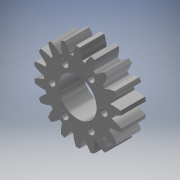
# Autodesk Inventor part: Цилиндрическое зубчатое зацепление2
Saved by Autodesk Inventor 2019 (Build 230136000, 136)
## iProperties
Created: 2020-03-13
Part Number: Цилиндрическое зубчатое зацепление2
Material: Steel
Document SubType Name: Modeling
Designer: Петров Иван
Categories: <?xml version="1.0" encoding="UTF-16"?> <MemberInstance><Categories><FamilyTemplate><FamilyTemplateParameter ValueType="xs:double" Id="1" ObjectReferenceKey="da_z" ObjectType="kUserParameterObject"/><FamilyTemplateParameter ValueType="xs:double" Id="2" ObjectReferenceKey="da_b" ObjectType="kUserParameterObject"/><FamilyTemplateParameter ValueType="xs:double" Id="3" ObjectReferenceKey="da_beta" ObjectType="kUserParameterObject"/><FamilyTemplateParameter ValueType="xs:double" Id="4" ObjectReferenceKey="da_da" ObjectType="kUserParameterObject"/><FamilyTemplateParameter ValueType="xs:double" Id="5" ObjectReferenceKey="da_aw" ObjectType="kUserParameterObject"/><FamilyTemplateParameter ValueType="xs:string" Id="6" ObjectReferenceKey="EAIAABAAAACIAQAAAAAAAIAAAAAAAAAA" ObjectType="83910656" SubObjectId="SurfaceGeometry"/></FamilyTemplate><ParamToTemplateMap><ParamToTemplate CategoryParameter="//CategoryParameter[@InternalName='046C89C9-8512-4d59-83FE-43B91F4F132A']" TemplateParameter="1"/><ParamToTemplate CategoryParameter="//CategoryParameter[@InternalName='2552DF32-E462-4b46-AEBF-C6C7768E72AC']" TemplateParameter="2"/><ParamToTemplate CategoryParameter="//CategoryParameter[@InternalName='C9EE641D-15FC-4fae-A226-E94C4372FDD7']" TemplateParameter="3"/><ParamToTemplate><ParamToTemplate CategoryParameter="//CategoryParameter[@InternalName='00B6519A-459B-49c7-AD84-2E56D39A5744']" ConstantValue="-0.108464"/></ParamToTemplate><ParamToTemplate><ParamToTemplate CategoryParameter="//CategoryParameter[@InternalName='04B31F0E-C7A6-4894-AA32-9629BEFACF47']" ConstantValue="1.000000"/></ParamToTemplate><ParamToTemplate><ParamToTemplate CategoryParameter="//CategoryParameter[@InternalName='43CBEC2E-7847-49e7-A936-2F7889FCB2D9']" ConstantValue="0.250000"/></ParamToTemplate><ParamToTemplate><ParamToTemplate CategoryParameter="//CategoryParameter[@InternalName='B1EFC894-105D-4ebd-86BF-FA20ED196853']" ConstantValue="0.350000"/></ParamToTemplate><ParamToTemplate><ParamToTemplate CategoryParameter="//CategoryParameter[@InternalName='51175063-3D10-4879-93E8-6246FE8B403D']" ConstantValue="2060000000.000000"/></ParamToTemplate><ParamToTemplate><ParamToTemplate CategoryParameter="//CategoryParameter[@InternalName='A3A52E27-4454-46a9-B0BD-C932399B70AF']" ConstantValue="0.300000"/></ParamToTemplate><ParamToTemplate><ParamToTemplate CategoryParameter="//CategoryParameter[@InternalName='91B76062-C214-41d9-B1B9-14D2AB99603D']" ConstantValue="0.090000"/></ParamToTemplate><ParamToTemplate><ParamToTemplate CategoryParameter="//CategoryParameter[@InternalName='374E806E-8B8A-4dda-A9AA-1039D6500AD2']" ConstantValue="11.111111"/></ParamToTemplate><ParamToTemplate><ParamToTemplate CategoryParameter="//CategoryParameter[@InternalName='2D373A89-B862-43d6-8D0B-0CBF12AB9F6C']" ConstantValue="0.349066"/></ParamToTemplate><ParamToTemplate CategoryParameter="//CategoryParameter[@InternalName='37777632-D6A2-4fac-9D53-DB8ACD95C989']" TemplateParameter="4"/><ParamToTemplate CategoryParameter="//CategoryParameter[@InternalName='FD1017F1-B727-4f7e-9707-0F86F1FF9423']" TemplateParameter="5"/><ParamToTemplate><ParamToTemplate CategoryParameter="//CategoryParameter[@InternalName='9E1B4470-B2D3-4ff1-B813-535BB4CDF51A']" ConstantValue="3520000.000000"/></ParamToTemplate><ParamToTemplate><ParamToTemplate CategoryParameter="//CategoryParameter[@InternalName='F8452263-BFF6-458c-9FB1-07C4B99E95CD']" ConstantValue="11400000.000000"/></ParamToTemplate><ParamToTemplate><ParamToTemplate CategoryParameter="//CategoryParameter[@InternalName='3E3BB259-FD49-497f-8171-6EBC954A3479']" ConstantValue="2.000000"/></ParamToTemplate><ParamToTemplate CategoryParameter="//CategoryParameter[@InternalName='27C3BAF2-7550-4e4b-AE2C-0DB134B7D9B7']" TemplateParameter="6"/></ParamToTemplateMap><Category DisplayName="Gear" InternalName="DC85795E-93AB-48d5-8EEE-5A27447B64BD" Mnemonic="Gear"><CategoryParameter DisplayName="z" InternalName="046C89C9-8512-4d59-83FE-43B91F4F132A" Mnemonic="z"/><CategoryParameter DisplayName="b" InternalName="2552DF32-E462-4b46-AEBF-C6C7768E72AC" Mnemonic="b"/><CategoryParameter DisplayName="||b|" InternalName="C9EE641D-15FC-4fae-A226-E94C4372FDD7" Mnemonic="beta"/><CategoryParameter DisplayName="x" InternalName="00B6519A-459B-49c7-AD84-2E56D39A5744" Mnemonic="x"/><CategoryParameter DisplayName="a*" InternalName="04B31F0E-C7A6-4894-AA32-9629BEFACF47" Mnemonic="a"/><CategoryParameter DisplayName="c*" InternalName="43CBEC2E-7847-49e7-A936-2F7889FCB2D9" Mnemonic="c"/><CategoryParameter DisplayName="r|.f|*" InternalName="B1EFC894-105D-4ebd-86BF-FA20ED196853" Mnemonic="rf"/><CategoryParameter DisplayName="E" InternalName="51175063-3D10-4879-93E8-6246FE8B403D" Mnemonic="E"/><CategoryParameter DisplayName="||m|" InternalName="A3A52E27-4454-46a9-B0BD-C932399B70AF" Mnemonic="mi"/><Category DisplayName="SpurGear" InternalName="26C5A22E-A91E-4dfd-A3B3-23CCAFAE1764" Mnemonic="SpurGear"><CategoryParameter DisplayName="m" InternalName="91B76062-C214-41d9-B1B9-14D2AB99603D" Mnemonic="m"/><CategoryParameter DisplayName="P" InternalName="374E806E-8B8A-4dda-A9AA-1039D6500AD2" Mnemonic="PP"/><CategoryParameter DisplayName="||a|" InternalName="2D373A89-B862-43d6-8D0B-0CBF12AB9F6C" Mnemonic="alpha"/><CategoryParameter DisplayName="d|.a|" InternalName="37777632-D6A2-4fac-9D53-DB8ACD95C989" Mnemonic="da"/><CategoryParameter DisplayName="a|.w|" InternalName="FD1017F1-B727-4f7e-9707-0F86F1FF9423" Mnemonic="aw"/><CategoryParameter DisplayName="||s||.Flim|" InternalName="9E1B4470-B2D3-4ff1-B813-535BB4CDF51A" Mnemonic="sFlim"/><CategoryParameter DisplayName="||s||.Hlim|" InternalName="F8452263-BFF6-458c-9FB1-07C4B99E95CD" Mnemonic="sHlim"/><CategoryParameter DisplayName="тип" InternalName="3E3BB259-FD49-497f-8171-6EBC954A3479" Mnemonic="type"/><CategoryParameter DisplayName="PitchDiameter" InternalName="27C3BAF2-7550-4e4b-AE2C-0DB134B7D9B7" Mnemonic="IDS_PITCHDIAM"/></Category></Category></Categories></MemberInstance>
Density: 1 g/cm^3
Appearance: Steel
CustomPartVersion: 1
Author: Петров Иван
Autodesk Inventor part; units mm, degrees
ref_plane "YZ Plane" through (0, 0, 0) normal (1, 0, 0) x (0, 1, 0)
ref_plane "XZ Plane" through (0, 0, 0) normal (0, 1, 0) x (-1, 0, 0)
ref_plane "XY Plane" through (0, 0, 0) normal (0, 0, 1) x (1, 0, 0)
sketch "Sketch1" plane through (0, 0, 0) normal (0, 0, 1) x (1, 0, 0)
  circle A0 centre (0, 0) radius 8.9
  dimension "d0" = 17.8
  constraints: 1 centre point
  measures "d0" diameter of A0
extrude "Extrusion1" add sketch "Sketch1" along normal blind 5
ref_plane "Work Plane2" through (0, 0, 2.5) normal (0, 0, 1) x (1, 0, 0)
sketch "Sketch2" plane through (0, 0, 0) normal (0, 0, -1) x (-1, 0, 0)
  circle A0 centre (0, 0) radius 8.9 projected
  circle A1 centre (0, 0) radius 8.05
  dimension "d3" = 16.1
  constraints: 1 centre point, 1 coincident
  measures "d3" diameter of A1
surface extrude "Средний диаметр" sketch "Sketch2" against normal through all shown no curves A1
ref_plane "Work Plane8" through (0, 0, 0) normal (0.9848078, 0.1736482, 0) x (0, 0, 1)
ref_plane "Work Plane9" through (0, 0, 0) normal (1, 0, 0) x (0, 1, 0)
spur gear teeth "Цилиндрическое зубчатое зацепление" teeth 18 pitch diameter 16.2 tip diameter 17.8 root diameter 13.7548 face width 5 start plane through (0, 0, 0) normal (0, 0, -1) x (-1, 0, 0)
sketch "Эскиз3" plane through (0, 0, 5) normal (0, 0, 1) x (1, 0, 0)
  circle A0 centre (0, 0) radius 3.85
  dimension "d49" = 7.7
  constraints: 1 centre point, 1 coincident
  measures "d49" diameter of A0
extrude "Выдавливание2" cut sketch "Эскиз3" against normal blind 12
sketch "Эскиз4" plane through (0, 0, 5) normal (0, 0, 1) x (1, 0, 0)
  line L0 (0, 0) -> (-5.3, 0)
  circle A0 centre (-5.3, 0) radius 0.75
  dimension "d52" = 5.3
  dimension "d53" = 1.5
  constraints: 2 end point, 1 centre point, 1 coincident, 1 horizontal
  measures "d52" distance of L0.start L0.end
  measures "d53" diameter of A0
extrude "Выдавливание3" cut sketch "Эскиз4" against normal blind 33.25
pattern_circular "Круговой массив1" count 6 over 360 about axis through (0, 0, 5) along (0, 0, -1) of "Выдавливание3"
sketch "Эскиз5" plane through (0, 0, 5) normal (0, 0, 1) x (1, 0, 0)
  circle A0 centre (-2.65, -4.5899) radius 0.75 projected
  circle A1 centre (2.65, -4.5899) radius 0.75 projected
  circle A2 centre (5.3, 0) radius 0.75 projected
  circle A3 centre (2.65, 4.5899) radius 0.75 projected
  circle A4 centre (-2.65, 4.5899) radius 0.75 projected
  circle A5 centre (-5.3, 0) radius 0.75 projected
  circle A6 centre (0, 0) radius 3.85 projected
  arc A7 (-3.4059, 8.2225) -> (-3.1756, 6.1003) centre (3.6513, 7.9146) ccw projected
  arc A8 (-3.1756, 6.1003) -> (-3.6952, 5.8003) centre (0, 0) ccw projected
  arc A9 (-3.6952, 5.8003) -> (-5.418, 7.0608) centre (-8.6799, 0.7952) ccw projected
  arc A10 (-5.418, 7.0608) -> (-6.0128, 6.5618) centre (0, 0) ccw projected
  arc A11 (-6.0128, 6.5618) -> (-5.0705, 4.6463) centre (0.7241, 8.6861) ccw projected
  arc A12 (-5.0705, 4.6463) -> (-5.4562, 4.1867) centre (0, 0) ccw projected
  arc A13 (-5.4562, 4.1867) -> (-7.5062, 4.782) centre (-8.4284, -2.2214) ccw projected
  arc A14 (-7.5062, 4.782) -> (-7.8944, 4.1096) centre (0, 0) ccw projected
  arc A15 (-7.8944, 4.1096) -> (-6.3539, 2.6319) centre (-2.2904, 8.4099) ccw projected
  arc A16 (-6.3539, 2.6319) -> (-6.5591, 2.0681) centre (0, 0) ccw projected
  arc A17 (-6.5591, 2.0681) -> (-8.689, 1.9263) centre (-7.1604, -4.9702) ccw projected
  arc A18 (-8.689, 1.9263) -> (-8.8239, 1.1617) centre (0, 0) ccw projected
  arc A19 (-8.8239, 1.1617) -> (-6.8708, 0.3) centre (-5.0286, 7.1194) ccw projected
  arc A20 (-6.8708, 0.3) -> (-6.8708, -0.3) centre (0, 0) ccw projected
  arc A21 (-6.8708, -0.3) -> (-8.8239, -1.1617) centre (-5.0286, -7.1194) ccw projected
  arc A22 (-8.8239, -1.1617) -> (-8.689, -1.9263) centre (0, 0) ccw projected
  arc A23 (-8.689, -1.9263) -> (-6.5591, -2.0681) centre (-7.1604, 4.9702) ccw projected
  arc A24 (-6.5591, -2.0681) -> (-6.3539, -2.6319) centre (0, 0) ccw projected
  arc A25 (-6.3539, -2.6319) -> (-7.8944, -4.1096) centre (-2.2904, -8.4099) ccw projected
  arc A26 (-7.8944, -4.1096) -> (-7.5062, -4.782) centre (0, 0) ccw projected
  arc A27 (-7.5062, -4.782) -> (-5.4562, -4.1867) centre (-8.4284, 2.2214) ccw projected
  arc A28 (-5.4562, -4.1867) -> (-5.0705, -4.6463) centre (0, 0) ccw projected
  arc A29 (-5.0705, -4.6463) -> (-6.0128, -6.5618) centre (0.7241, -8.6861) ccw projected
  arc A30 (-6.0128, -6.5618) -> (-5.418, -7.0608) centre (0, 0) ccw projected
  arc A31 (-5.418, -7.0608) -> (-3.6952, -5.8003) centre (-8.6799, -0.7952) ccw projected
  arc A32 (-3.6952, -5.8003) -> (-3.1756, -6.1003) centre (0, 0) ccw projected
  arc A33 (-3.1756, -6.1003) -> (-3.4059, -8.2225) centre (3.6513, -7.9146) ccw projected
  arc A34 (-3.4059, -8.2225) -> (-2.6763, -8.4881) centre (0, 0) ccw projected
  arc A35 (-2.6763, -8.4881) -> (-1.4885, -6.7144) centre (-7.8845, -3.716) ccw projected
  arc A36 (-1.4885, -6.7144) -> (-0.8977, -6.8185) centre (0, 0) ccw projected
  arc A37 (-0.8977, -6.8185) -> (-0.3882, -8.8915) centre (6.138, -6.1885) ccw projected
  arc A38 (-0.3882, -8.8915) -> (0.3882, -8.8915) centre (0, 0) ccw projected
  arc A39 (0.3882, -8.8915) -> (0.8977, -6.8185) centre (-6.138, -6.1885) ccw projected
  arc A40 (0.8977, -6.8185) -> (1.4885, -6.7144) centre (0, 0) ccw projected
  arc A41 (1.4885, -6.7144) -> (2.6763, -8.4881) centre (7.8845, -3.716) ccw projected
  arc A42 (2.6763, -8.4881) -> (3.4059, -8.2225) centre (0, 0) ccw projected
  arc A43 (3.4059, -8.2225) -> (3.1756, -6.1003) centre (-3.6513, -7.9146) ccw projected
  arc A44 (3.1756, -6.1003) -> (3.6952, -5.8003) centre (0, 0) ccw projected
  arc A45 (3.6952, -5.8003) -> (5.418, -7.0608) centre (8.6799, -0.7952) ccw projected
  arc A46 (5.418, -7.0608) -> (6.0128, -6.5618) centre (0, 0) ccw projected
  arc A47 (6.0128, -6.5618) -> (5.0705, -4.6463) centre (-0.7241, -8.6861) ccw projected
  arc A48 (5.0705, -4.6463) -> (5.4562, -4.1867) centre (0, 0) ccw projected
  arc A49 (5.4562, -4.1867) -> (7.5062, -4.782) centre (8.4284, 2.2214) ccw projected
  arc A50 (7.5062, -4.782) -> (7.8944, -4.1096) centre (0, 0) ccw projected
  arc A51 (7.8944, -4.1096) -> (6.3539, -2.6319) centre (2.2904, -8.4099) ccw projected
  arc A52 (6.3539, -2.6319) -> (6.5591, -2.0681) centre (0, 0) ccw projected
  arc A53 (6.5591, -2.0681) -> (8.689, -1.9263) centre (7.1604, 4.9702) ccw projected
  arc A54 (8.689, -1.9263) -> (8.8239, -1.1617) centre (0, 0) ccw projected
  arc A55 (8.8239, -1.1617) -> (6.8708, -0.3) centre (5.0286, -7.1194) ccw projected
  arc A56 (6.8708, -0.3) -> (6.8708, 0.3) centre (0, 0) ccw projected
  arc A57 (6.8708, 0.3) -> (8.8239, 1.1617) centre (5.0286, 7.1194) ccw projected
  arc A58 (8.8239, 1.1617) -> (8.689, 1.9263) centre (0, 0) ccw projected
  arc A59 (8.689, 1.9263) -> (6.5591, 2.0681) centre (7.1604, -4.9702) ccw projected
  arc A60 (6.5591, 2.0681) -> (6.3539, 2.6319) centre (0, 0) ccw projected
  arc A61 (6.3539, 2.6319) -> (7.8944, 4.1096) centre (2.2904, 8.4099) ccw projected
  arc A62 (7.8944, 4.1096) -> (7.5062, 4.782) centre (0, 0) ccw projected
  arc A63 (7.5062, 4.782) -> (5.4562, 4.1867) centre (8.4284, -2.2214) ccw projected
  arc A64 (5.4562, 4.1867) -> (5.0705, 4.6463) centre (0, 0) ccw projected
  arc A65 (5.0705, 4.6463) -> (6.0128, 6.5618) centre (-0.7241, 8.6861) ccw projected
  arc A66 (6.0128, 6.5618) -> (5.418, 7.0608) centre (0, 0) ccw projected
  arc A67 (5.418, 7.0608) -> (3.6952, 5.8003) centre (8.6799, 0.7952) ccw projected
  arc A68 (3.6952, 5.8003) -> (3.1756, 6.1003) centre (0, 0) ccw projected
  arc A69 (3.1756, 6.1003) -> (3.4059, 8.2225) centre (-3.6513, 7.9146) ccw projected
  arc A70 (3.4059, 8.2225) -> (2.6763, 8.4881) centre (0, 0) ccw projected
  arc A71 (2.6763, 8.4881) -> (1.4885, 6.7144) centre (7.8845, 3.716) ccw projected
  arc A72 (1.4885, 6.7144) -> (0.8977, 6.8185) centre (0, 0) ccw projected
  arc A73 (0.8977, 6.8185) -> (0.3882, 8.8915) centre (-6.138, 6.1885) ccw projected
  arc A74 (0.3882, 8.8915) -> (-0.3882, 8.8915) centre (0, 0) ccw projected
  arc A75 (-0.3882, 8.8915) -> (-0.8977, 6.8185) centre (6.138, 6.1885) ccw projected
  arc A76 (-0.8977, 6.8185) -> (-1.4885, 6.7144) centre (0, 0) ccw projected
  arc A77 (-1.4885, 6.7144) -> (-2.6763, 8.4881) centre (-7.8845, 3.716) ccw projected
  arc A78 (-2.6763, 8.4881) -> (-3.4059, 8.2225) centre (0, 0) ccw projected
equation "\"d0\" = da_da"
equation "\"d1\" = da_b"
equation "\"d3\" = da_dw"
equation "\"d16\" = da_aw"
equation "\"d43\" = da_aw"
equation "\"d46\" = da_aw"
equation "\"da_da\" = 17.8"
equation "\"da_b\" = 5"
equation "\"da_dw\" = 16.1"
equation "\"da_aw\" = 16.1"
body "Solid1"
body "Srf1"
